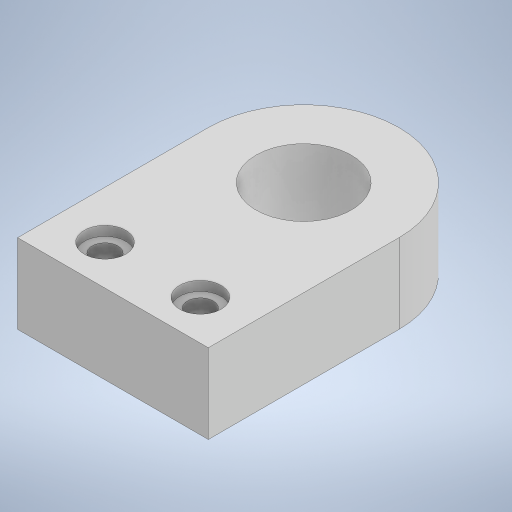
# Autodesk Inventor part: element3_obj4
Saved by Autodesk Inventor 2023.2 (Build 272271030, 271C)
## iProperties
Created: 2023-02-25
Part Number: element3_obj4
Material: Generic
Document SubType Name: Modeling
Designer: Cris Pat
Density: 1 g/cm^3
Appearance: Default
Author: Cris Pat
Autodesk Inventor part; units mm, degrees
ref_plane "YZ Plane" through (0, 0, 0) normal (1, 0, 0) x (0, 1, 0)
ref_plane "XZ Plane" through (0, 0, 0) normal (0, 1, 0) x (-1, 0, 0)
ref_plane "XY Plane" through (0, 0, 0) normal (0, 0, 1) x (1, 0, 0)
sketch "Sketch1" plane through (0, 0, 0) normal (0, 1, 0) x (-1, 0, 0)
  line L0 (30, 60) -> (-30, 60)
  line L1 (-30, 60) -> (-30, 0)
  arc A0 (-30, 0) -> (30, 0) centre (0, 0) ccw
  line L2 (30, 0) -> (30, 60)
  circle A1 centre (0, 0) radius 15
  dimension "d0" = 60
  dimension "d1" = 60
  dimension "d2" = 30
  constraints: 6 end point, 3 coincident, 2 centre point, 2 point on circle, 2 tangent, 1 horizontal, 1 parallel, 1 perpendicular
  measures "d0" distance of L0.start L0.end
  measures "d1" distance of L0.end L1.end
  measures "d2" diameter of A1
extrude "Extrusion1" add sketch "Sketch1" along normal mid plane 25
sketch "Sketch2" plane through (0, 0, 0) normal (0, 1, 0) x (-1, 0, 0)
  line L0 (-30, 0) -> (-30, 60) construction
  line L1 (-30, 60) -> (30, 60) construction
  line L2 (30, 60) -> (30, 0) construction
  arc A0 (-30, 0) -> (30, 0) centre (0, 0) ccw construction
  circle A1 centre (0, 0) radius 15 construction
  line L3 (30, 60) -> (30, 0) construction
  line L4 (30, 35) -> (-30, 35) construction
  circle A2 centre (15, 47.5) radius 4.05
  line L5 (0, 35) -> (0, 60) construction
  circle A3 centre (-15, 47.5) radius 4.05
  point P0 (0, -30)
  point P1 (0, 47.5)
  dimension "d5" = 65
  dimension "d6" = 8.1
  dimension "d7" = 30
  constraints: 4 end point, 3 midpoint, 2 centre point, 2 point on line, 1 horizontal, 1 horizontal alignment, 1 point on circle, 1 symmetric about line, 1 other
  measures "d5" distance of L5.start point (0, -30)
  measures "d6" diameter of A2
  measures "d7" distance of A3.centre A2.centre
extrude "Extrusion2" cut sketch "Sketch2" along normal through all both and the other way through all
sketch "Sketch3" plane through (0, 12.5, 0) normal (0, 1, 0) x (1, 0, 0)
  circle A0 centre (-15, -47.5) radius 4.05 construction
  circle A1 centre (15, -47.5) radius 4.05 construction
  line L0 (30, -60) -> (30, 0) construction
  arc A2 (30, 0) -> (-30, 0) centre (0, 0) ccw construction
  line L1 (-30, 0) -> (-30, -60) construction
  line L2 (-30, -60) -> (30, -60) construction
  circle A3 centre (0, 0) radius 15 construction
  circle A4 centre (-15, -47.5) radius 4.05 projected
  circle A5 centre (-15, -47.5) radius 6.55
  circle A6 centre (15, -47.5) radius 6.55
  dimension "d10" = 13.1
  dimension "d11" = 13.1
  constraints: 2 centre point, 2 coincident
  measures "d10" diameter of A5
  measures "d11" diameter of A6
extrude "Extrusion3" cut sketch "Sketch3" against normal blind 3 contours A4 | A5 | A6
body "Solid1"
